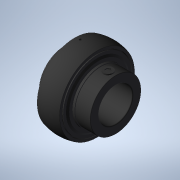
# Autodesk Inventor part: YAR 205-014-2F-33.740-b
Saved by Autodesk Inventor 2021 (Build 250183000, 183)
## iProperties
Created: 2025-11-05
Part Number: YAR 205-014-2F-33.740-b
Material: Generic
Catalog Web Link: www.3dfindit.com
Description: ayp_001_hc_hh_hy-ayl_001_hp_bearing-Y-bearings
Vendor: SKF
Document SubType Name: Modeling
Designer: psAdmin
Manufacturer: SKF
Mass: 220 g
Surface Area: 222.201 cm^2
Volume: 25.7609 cm^3
Density: 1 g/cm^3
Appearance: PSOLRGB-176-176-176
Category: PARTsolutions
Company: SKF
Title: YAR 205-014-2F-33.740-b
Author: Cadenas PARTsolutions
Comments: Y-bearings
PSOL_IDENT_0: {$CADENAS_DATA/23d-libs/skf/bearings_units_and_housings/bearing_units/ball_bearing_units/y-units/y-b
PSOL_IDENT_1: earing_plummer_block_units_parts/ayp_001_hc_hh_hy-ayl_001_hp_bearing.prj},217 {VTYP=3D},{NB=YAR 205-
PSOL_IDENT_2: 014-2F-33.740-b},{LINA=YAR 205-014-2F-33.740-b},{NN=ayp_001_hc_hh_hy-ayl_001_hp_bearing},{DATE=14.11
PSOL_IDENT_3: .2022 08:30:30},{GEOMDATE=05.09.2022 08:59:11},{VERSION=},{LINEID=3080},{WBVAR=},{WBNUMERIC=}  {NB=Y
PSOL_IDENT_4: AR 205-014-2F-33.740-b},{LINA=YAR 205-014-2F-33.740-b},{KT=DUMMY},{PRODUCTID=0},{DESIGNATION=YAR 205
PSOL_IDENT_5: -014-2F},{DD=22.2250},{D=52},{B=34.100},{C=15.000},{PITCH=39.040},{DW=7.938},{FO=IEC_BBY_006},{DESIG
PSOL_IDENT_6: N=ybrg1},{SLEEVE=},{B1=MIN},{LM=Grub screw},{DES=Inner ring extended on both sides},{PS=For agricult
PSOL_IDENT_7: ural applications},{MAT=},{SS=Standard seals with additional flingers},{UNIT=Inch},{G=MIN},{DD1=33.7
PSOL_IDENT_8: 4},{DD2=MIN},{DD3=MIN},{B3=0.000},{B4=MIN},{BB4=5.0},{R12=0.6},{R12X=0},{SS1=19.800},{NOTE=},{DG=MIN
PSOL_IDENT_9: },{E=4.350},{F=1.700},{RG=MIN},{LOAD1=14.000},{LOAD2=7.800},{LOAD3=0.335},{SPEED2=7000},{FF0=14},{BF=
PSOL_IDENT_10: 1},{A15=500000},{A8=400000},{A4=300000},{BETA=1.89},{SBT1=0.094},{SBT2=},{RF1=0.00000039},{RF2=1.7},
PSOL_IDENT_11: {SF1=0.00323},{SF2=36.5},{KZ=3.1},{II=1},{Z=9},{SG=VT307},{MASS=0.22},{G2=1/4-28 UNF},{HEX=3.175},{R
PSOL_IDENT_12: TT=4},{MKIT=},{AS=},{TANGLE=},{SRING=RIS 205},{FPC=},{POPI=1},{NOUN=N020},{NOUNDES=Ball bearing},{MO
PSOL_IDENT_13: D=M200},{MODDES=Radial deep groove},{YZ=16.87},{PIM=YAR 205-014-2F},{LNDD11=MIN},{LUB3=0},{BZ=0.4708
PSOL_IDENT_14: },{SDALG=h},{YRZ=23.489},{SHAPE=4},{LNB1HM11=0},{LWM=0},{TYPEID=0},{LUBGR2=0},{LOCKNUT=},{LOCKDEVICE=
PSOL_IDENT_15: },{LNB=MIN},{BB=MIN},{LNB1=MIN},{S1ALG=19.8},{HH=MIN},{LDB=MIN},{LDDD1=MIN},{LDDD2=MIN},{LDM=MIN},{L
PSOL_IDENT_16: DFF=MIN},{TP=4},{LNBHM11=0},{BBHM11=0},{LNDD1HM11=0},{HELP=5},{HHHM11=0},{LUBGR1=0},{LWV=0},{S2=26},
PSOL_IDENT_17: {LUB2=0},{BZ1=0.000},{HEX2=}
NB: YAR 205-014-2F-33.740-b
NN: ayp_001_hc_hh_hy-ayl_001_hp_bearing
NT: Y-bearings
NBSYN: $DESIGNATION.-$DD1.$PRODUCTID.-b
LINA: YAR 205-014-2F-33.740-b
CATALOG: SKF
DESIGNATION: YAR 205-014-2F
DD: 22.225
D: 52
B: 34.1
C: 15
B1: 0
DD1: 33.74
LOAD1: 14
LOAD2: 7.8
LOAD3: 0.335
SPEED2: 7000
SUPPLIER: SKF
ARTICLENO: YAR 205-014-2F-33.740-b
BOMINFO: YAR 205-014-2F-33.740-b
CREATOR: CADENAS GmbH
Autodesk Inventor part; units mm, degrees
sketch "Sketch_1" plane through (0, 0, 0) normal (0, 0, 1) x (1, 0, 0)
  line L0 (50, 0) -> (-50, 0)
  line L1 (-14.3, 16.57) -> (-14.3, 11.7125)
  arc A0 (-14.3, 11.7125) -> (-13.7, 11.1125) centre (-13.7, 11.7125) ccw
  line L2 (-13.7, 11.1125) -> (19.2, 11.1125)
  arc A1 (19.2, 11.1125) -> (19.8, 11.7125) centre (19.2, 11.7125) ccw
  line L3 (19.8, 11.7125) -> (19.8, 16.57)
  arc A2 (19.8, 16.57) -> (19.5, 16.87) centre (19.5, 16.57) ccw
  line L4 (19.5, 16.87) -> (2.9547, 16.87)
  arc A3 (-2.9547, 16.87) -> (2.9547, 16.87) centre (0, 19.52) ccw
  line L5 (-2.9547, 16.87) -> (-14, 16.87)
  arc A4 (-14, 16.87) -> (-14.3, 16.57) centre (-14, 16.57) ccw
  constraints: 12 end point, 10 point on circle, 5 centre point
revolve "Revolution1" add sketch "Sketch_1" angle 360 about axis through (50, 0, 0) along (1, 0, 0)
sketch "Sketch_2" plane through (0, 11.1125, 0) normal (0, 1, 0) x (1, 0, 0)
  circle A0 centre (14.8, 0) radius 3.175
  line L0 (13.2125, -0.9165) -> (14.8, -1.8331)
  line L1 (14.8, -1.8331) -> (16.3875, -0.9165)
  line L2 (16.3875, -0.9165) -> (16.3875, 0.9165)
  line L3 (16.3875, 0.9165) -> (14.8, 1.8331)
  line L4 (14.8, 1.8331) -> (13.2125, 0.9165)
  line L5 (13.2125, 0.9165) -> (13.2125, -0.9165)
  constraints: 12 end point, 1 centre point
extrude "Extrusion1" add sketch "Sketch_2" along normal blind 6.3333
sketch "Sketch_3" plane through (0, -5.5563, -9.6237) normal (0, -0.5, -0.866) x (1, 0, 0)
  circle A0 centre (14.8, 0) radius 3.175
  line L0 (13.2125, -0.9165) -> (14.8, -1.8331)
  line L1 (14.8, -1.8331) -> (16.3875, -0.9165)
  line L2 (16.3875, -0.9165) -> (16.3875, 0.9165)
  line L3 (16.3875, 0.9165) -> (14.8, 1.8331)
  line L4 (14.8, 1.8331) -> (13.2125, 0.9165)
  line L5 (13.2125, 0.9165) -> (13.2125, -0.9165)
  constraints: 12 end point, 1 centre point
extrude "Extrusion2" add sketch "Sketch_3" along normal blind 6.3333
sketch "Sketch_4" plane through (0, 0, 0) normal (0, 0, 1) x (1, 0, 0)
  line L0 (7.5, 0) -> (-7.5, 0)
  line L1 (-9.877, 17.3408) -> (-9.877, 16.87)
  line L2 (-9.877, 16.87) -> (-7.9938, 16.87)
  line L3 (-7.9938, 16.87) -> (-7.9938, 19.52)
  line L4 (-7.9938, 19.52) -> (-7.2646, 20.843)
  line L5 (-7.2646, 20.843) -> (-7.2646, 22.7536)
  line L6 (-7.2646, 22.7536) -> (-7.7354, 22.7536)
  line L7 (-7.7354, 22.7536) -> (-7.7354, 20.843)
  line L8 (-7.7354, 20.843) -> (-8.4646, 19.52)
  line L9 (-8.4646, 19.52) -> (-8.4646, 17.3408)
  line L10 (-8.4646, 17.3408) -> (-9.877, 17.3408)
  constraints: 22 end point
revolve "Revolution2" add sketch "Sketch_4" angle 360 about axis through (7.5, 0, 0) along (1, 0, 0)
sketch "Sketch_5" plane through (0, 0, 0) normal (0, 0, 1) x (1, 0, 0)
  line L0 (7.5, 0) -> (-7.5, 0)
  line L1 (7.2646, 22.7536) -> (7.2646, 20.843)
  line L2 (7.2646, 20.843) -> (7.9938, 19.52)
  line L3 (7.9938, 19.52) -> (7.9938, 16.87)
  line L4 (7.9938, 16.87) -> (9.877, 16.87)
  line L5 (9.877, 16.87) -> (9.877, 17.3408)
  line L6 (9.877, 17.3408) -> (8.4646, 17.3408)
  line L7 (8.4646, 17.3408) -> (8.4646, 19.52)
  line L8 (8.4646, 19.52) -> (7.7354, 20.843)
  line L9 (7.7354, 20.843) -> (7.7354, 22.7536)
  line L10 (7.7354, 22.7536) -> (7.2646, 22.7536)
  constraints: 22 end point
revolve "Revolution3" add sketch "Sketch_5" angle 360 about axis through (7.5, 0, 0) along (1, 0, 0)
sketch "Sketch_6" plane through (0, 0, 0) normal (0, 0, 1) x (1, 0, 0)
  line L0 (50, 0) -> (-50, 0)
  line L1 (-7.5, 19.9606) -> (-7.5, 17.2671)
  line L2 (-7.5, 17.2671) -> (-7.0292, 17.2671)
  line L3 (-7.0292, 17.2671) -> (-7.0292, 19.7138)
  line L4 (-7.0292, 19.7138) -> (-5.0717, 21.0682)
  line L5 (-5.0717, 21.0682) -> (-5.0181, 20.9908)
  line L6 (-5.0181, 20.9908) -> (-6.935, 19.6644)
  line L7 (-6.935, 19.6644) -> (-6.935, 17.4657)
  line L8 (-6.935, 17.4657) -> (-5.1617, 17.4657)
  line L9 (-5.1617, 17.4657) -> (-5.3029, 16.87)
  line L10 (-5.3029, 16.87) -> (-4.8321, 16.87)
  line L11 (-4.8321, 16.87) -> (-4.6752, 17.5319)
  line L12 (-4.6752, 17.5319) -> (-4.6752, 18.1938)
  line L13 (-4.6752, 18.1938) -> (-5.3029, 18.8557)
  line L14 (-5.3029, 18.8557) -> (-5.3029, 20.1795)
  line L15 (-5.3029, 20.1795) -> (-4.6752, 20.8414)
  line L16 (-4.6752, 20.8414) -> (-4.6752, 23.3321)
  arc A0 (-4.6752, 23.3321) -> (-4.8321, 23.489) centre (-4.8321, 23.3321) ccw
  line L17 (-4.8321, 23.489) -> (-4.9891, 23.489)
  arc A1 (-4.9891, 23.489) -> (-5.146, 23.3321) centre (-4.9891, 23.3321) ccw
  line L18 (-5.146, 23.3321) -> (-5.9775, 22.3412)
  line L19 (-5.9775, 22.3412) -> (-5.6168, 22.0386)
  line L20 (-5.6168, 22.0386) -> (-5.146, 22.5996)
  line L21 (-5.146, 22.5996) -> (-5.146, 21.5893)
  line L22 (-5.146, 21.5893) -> (-7.5, 19.9606)
  constraints: 46 end point, 4 point on circle, 2 centre point
revolve "Revolution4" add sketch "Sketch_6" angle 360 about axis through (50, 0, 0) along (1, 0, 0)
sketch "Sketch_11" plane through (0, 0, 0) normal (0, 0, 1) x (1, 0, 0)
  line L0 (50, 0) -> (-50, 0)
  line L1 (4.6752, 23.3321) -> (4.6752, 20.8414)
  line L2 (4.6752, 20.8414) -> (5.3029, 20.1795)
  line L3 (5.3029, 20.1795) -> (5.3029, 18.8557)
  line L4 (5.3029, 18.8557) -> (4.6752, 18.1938)
  line L5 (4.6752, 18.1938) -> (4.6752, 17.5319)
  line L6 (4.6752, 17.5319) -> (4.8321, 16.87)
  line L7 (4.8321, 16.87) -> (5.3029, 16.87)
  line L8 (5.3029, 16.87) -> (5.1617, 17.4657)
  line L9 (5.1617, 17.4657) -> (6.935, 17.4657)
  line L10 (6.935, 17.4657) -> (6.935, 19.6644)
  line L11 (6.935, 19.6644) -> (5.0181, 20.9908)
  line L12 (5.0181, 20.9908) -> (5.0717, 21.0682)
  line L13 (5.0717, 21.0682) -> (7.0292, 19.7138)
  line L14 (7.0292, 19.7138) -> (7.0292, 17.2671)
  line L15 (7.0292, 17.2671) -> (7.5, 17.2671)
  line L16 (7.5, 17.2671) -> (7.5, 19.9606)
  line L17 (7.5, 19.9606) -> (5.146, 21.5893)
  line L18 (5.146, 21.5893) -> (5.146, 22.5996)
  line L19 (5.146, 22.5996) -> (5.6168, 22.0386)
  line L20 (5.6168, 22.0386) -> (5.9775, 22.3412)
  line L21 (5.9775, 22.3412) -> (5.146, 23.3321)
  arc A0 (5.146, 23.3321) -> (4.9891, 23.489) centre (4.9891, 23.3321) ccw
  line L22 (4.9891, 23.489) -> (4.8321, 23.489)
  arc A1 (4.8321, 23.489) -> (4.6752, 23.3321) centre (4.8321, 23.3321) ccw
  constraints: 46 end point, 4 point on circle, 2 centre point
revolve "Revolution5" add sketch "Sketch_11" angle 360 about axis through (50, 0, 0) along (1, 0, 0)
sketch "Sketch_16" plane through (0, 0, 0) normal (0, 0, 1) x (1, 0, 0)
  line L0 (7.5, 0) -> (-7.5, 0)
  line L1 (-7.5, 23.2786) -> (-5.2395, 23.2786)
  line L2 (-5.2395, 23.2786) -> (-5.0722, 23.4199)
  arc A0 (-4.6666, 23.2848) -> (-5.0722, 23.4199) centre (-4.9106, 23.2286) ccw
  line L3 (-4.6666, 23.2848) -> (-4.5761, 22.8921)
  arc A1 (-4.5761, 22.8921) -> (-4.3286, 22.6952) centre (-4.3286, 22.9492) ccw
  line L4 (-4.3286, 22.6952) -> (-2.4646, 22.6952)
  arc A2 (-2.4646, 22.6952) -> (-2.3164, 22.7429) centre (-2.4646, 22.9492) ccw
  arc A3 (2.3164, 22.7429) -> (-2.3164, 22.7429) centre (0, 19.52) ccw
  arc A4 (2.3164, 22.7429) -> (2.4646, 22.6952) centre (2.4646, 22.9492) ccw
  line L5 (2.4646, 22.6952) -> (4.3286, 22.6952)
  arc A5 (4.3286, 22.6952) -> (4.5761, 22.8921) centre (4.3286, 22.9492) ccw
  line L6 (4.5761, 22.8921) -> (4.6666, 23.2848)
  arc A6 (5.0722, 23.4199) -> (4.6666, 23.2848) centre (4.9106, 23.2286) ccw
  line L7 (5.0722, 23.4199) -> (5.2395, 23.2786)
  line L8 (5.2395, 23.2786) -> (7.5, 23.2786)
  line L9 (7.5, 23.2786) -> (7.5, 24.7457)
  arc A7 (7.5, 24.7457) -> (7.3566, 24.9375) centre (7.3, 24.7457) ccw
  arc A8 (7.3566, 24.9375) -> (-7.3566, 24.9375) centre (0, 0) ccw
  arc A9 (-7.3566, 24.9375) -> (-7.5, 24.7457) centre (-7.3, 24.7457) ccw
  line L10 (-7.5, 24.7457) -> (-7.5, 23.2786)
  constraints: 22 end point, 20 point on circle, 10 centre point
revolve "Revolution6" add sketch "Sketch_16" angle 360 about axis through (7.5, 0, 0) along (1, 0, 0)
sketch "Sketch_21" plane through (0, 0, 0) normal (0, 0, 1) x (1, 0, 0)
  line L0 (-3.5562, 19.52) -> (-3.5562, 39.04)
  line L1 (-3.5562, 39.04) -> (-2.7062, 39.04)
  line L2 (-2.7062, 39.04) -> (-2.7062, 19.52)
  line L3 (-2.7062, 19.52) -> (-3.5562, 19.52)
  line L4 (-3.5562, 19.52) -> (-3.5562, 39.04)
  constraints: 10 end point
revolve "Revolution7" cut sketch "Sketch_21" angle 360 about axis through (-3.5562, 19.52, 0) along (0, -1, 0)
ref_plane "ball_1_XY" through (0, 19.52, 0) normal (1, 0, 0) x (0, 0, -1)
ref_plane "ball_1_YZ" through (0, 19.52, 0) normal (0, 0, -1) x (0, 1, 0)
ref_plane "ball_1_ZX" through (0, 19.52, 0) normal (0, 1, 0) x (1, 0, 0)
ref_plane "ball_2_XY" through (0, 14.9532, 12.5472) normal (1, 0, 0) x (0, 0, -1)
ref_plane "ball_2_YZ" through (0, 14.9532, 12.5472) normal (0, 0, -1) x (0, 1, 0)
ref_plane "ball_2_ZX" through (0, 14.9532, 12.5472) normal (0, 1, 0) x (1, 0, 0)
ref_plane "ball_3_XY" through (0, 3.3896, 19.2234) normal (1, 0, 0) x (0, 0, -1)
ref_plane "ball_3_YZ" through (0, 3.3896, 19.2234) normal (0, 0, -1) x (0, 1, 0)
ref_plane "ball_3_ZX" through (0, 3.3896, 19.2234) normal (0, 1, 0) x (1, 0, 0)
ref_plane "ball_4_XY" through (0, -9.76, 16.9048) normal (1, 0, 0) x (0, 0, -1)
ref_plane "ball_4_YZ" through (0, -9.76, 16.9048) normal (0, 0, -1) x (0, 1, 0)
ref_plane "ball_4_ZX" through (0, -9.76, 16.9048) normal (0, 1, 0) x (1, 0, 0)
ref_plane "ball_5_XY" through (0, -18.3428, 6.6762) normal (1, 0, 0) x (0, 0, -1)
ref_plane "ball_5_YZ" through (0, -18.3428, 6.6762) normal (0, 0, -1) x (0, 1, 0)
ref_plane "ball_5_ZX" through (0, -18.3428, 6.6762) normal (0, 1, 0) x (1, 0, 0)
ref_plane "ball_6_XY" through (0, -18.3428, -6.6762) normal (1, 0, 0) x (0, 0, -1)
ref_plane "ball_6_YZ" through (0, -18.3428, -6.6762) normal (0, 0, -1) x (0, 1, 0)
ref_plane "ball_6_ZX" through (0, -18.3428, -6.6762) normal (0, 1, 0) x (1, 0, 0)
ref_plane "ball_7_XY" through (0, -9.76, -16.9048) normal (1, 0, 0) x (0, 0, -1)
ref_plane "ball_7_YZ" through (0, -9.76, -16.9048) normal (0, 0, -1) x (0, 1, 0)
ref_plane "ball_7_ZX" through (0, -9.76, -16.9048) normal (0, 1, 0) x (1, 0, 0)
ref_plane "ball_8_XY" through (0, 3.3896, -19.2234) normal (1, 0, 0) x (0, 0, -1)
ref_plane "ball_8_YZ" through (0, 3.3896, -19.2234) normal (0, 0, -1) x (0, 1, 0)
ref_plane "ball_8_ZX" through (0, 3.3896, -19.2234) normal (0, 1, 0) x (1, 0, 0)
ref_plane "ball_9_XY" through (0, 14.9532, -12.5472) normal (1, 0, 0) x (0, 0, -1)
ref_plane "ball_9_YZ" through (0, 14.9532, -12.5472) normal (0, 0, -1) x (0, 1, 0)
ref_plane "ball_9_ZX" through (0, 14.9532, -12.5472) normal (0, 1, 0) x (1, 0, 0)
ref_plane "brg_XY" through (0, 0, 0) normal (1, 0, 0) x (0, 0, -1)
ref_plane "brg_YZ" through (0, 0, 0) normal (0, 0, -1) x (0, 1, 0)
ref_plane "brg_ZX" through (0, 0, 0) normal (0, 1, 0) x (1, 0, 0)
body "Solid1"
